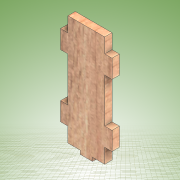
# Autodesk Inventor part: Caja_CaraFrontal
Saved by Autodesk Inventor 2022 (Build 260153000, 153)
## iProperties
Created: 2022-03-02
Part Number: Caja_CaraFrontal
Material: Genérico
Document SubType Name: Modeling
Designer: Marco
Density: 1 g/cm^3
Appearance: Valor por defecto
Author: Marco
Autodesk Inventor part; units mm, degrees
ref_plane "YZ Plane" through (0, 0, 0) normal (1, 0, 0) x (0, 1, 0)
ref_plane "XZ Plane" through (0, 0, 0) normal (0, 1, 0) x (-1, 0, 0)
ref_plane "XY Plane" through (0, 0, 0) normal (0, 0, 1) x (1, 0, 0)
sketch "Boceto1" plane through (0, 0, 0) normal (0, 0, 1) x (1, 0, 0)
  line L0 (0, 0) -> (30, 0)
  line L1 (30, 0) -> (30, 90)
  line L2 (30, 90) -> (0, 90)
  line L3 (0, 90) -> (0, 0)
  line L4 (30, 78) -> (36, 78)
  line L5 (36, 78) -> (36, 63)
  line L6 (36, 63) -> (30, 63)
  line L7 (30, 63) -> (30, 78)
  line L8 (30, 45) -> (0, 45) construction
  line L9 (30, 12) -> (36, 12)
  line L10 (36, 12) -> (36, 27)
  line L11 (36, 27) -> (30, 27)
  line L12 (30, 27) -> (30, 12)
  line L13 (15, 90) -> (15, 45) construction
  line L14 (0, 78) -> (-6, 78)
  line L15 (-6, 78) -> (-6, 63)
  line L16 (-6, 63) -> (0, 63)
  line L17 (0, 63) -> (0, 78)
  line L18 (0, 12) -> (-6, 12)
  line L19 (-6, 12) -> (-6, 27)
  line L20 (-6, 27) -> (0, 27)
  line L21 (0, 27) -> (0, 12)
  point P0 (30, 12)
  point P1 (30, 27)
  point P2 (30, 63)
  dimension "d0" = 30
  dimension "d1" = 90
  dimension "d2" = 6
  dimension "d3" = 15
  dimension "d4" = 12
  constraints: 44 end point, 12 symmetric about line, 4 midpoint, 4 parallel, 2 horizontal, 2 perpendicular, 1 point on line
  measures "d0" distance of L2.end L1.end
  measures "d1" distance of L2.end L0.start
  measures "d2" distance of L5.end L6.end
  measures "d3" distance of L4.end L5.end
  measures "d4" distance of L4.start L1.end
extrude "Extrusión1" add sketch "Boceto1" along normal blind 6
sketch "Boceto3" plane through (0, 0, 0) normal (0, -1, 0) x (1, 0, 0)
  line L0 (30, 6) -> (0, 6) projected
  line L1 (30, 0) -> (0, 0) projected
  line L2 (10, 6) -> (20, 6)
  line L3 (20, 6) -> (20, 0)
  line L4 (20, 0) -> (10, 0)
  line L5 (10, 0) -> (10, 6)
  point P0 (15, 6)
  point P1 (15, 6)
  dimension "d11" = 10
  constraints: 8 end point, 2 midpoint, 2 parallel, 2 point on line, 1 coincident, 1 horizontal, 1 perpendicular
  measures "d11" distance of L3.end L4.end
extrude "Extrusión3" add sketch "Boceto3" along normal blind 3
